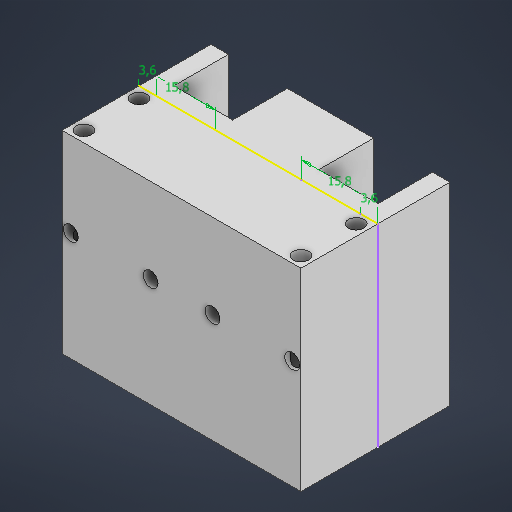
# Autodesk Inventor part: peça2
Saved by Autodesk Inventor 2026 (Build 300175000, 175)
## iProperties
Created: 2026-04-17
Part Number: peça2
Material: Genérico
Document SubType Name: Modeling
Designer: a2453266
Density: 1 g/cm^3
Appearance: Padrão
Author: a2453266
Autodesk Inventor part; units mm, degrees
ref_plane "YZ Plane" through (0, 0, 0) normal (1, 0, 0) x (0, 1, 0)
ref_plane "XZ Plane" through (0, 0, 0) normal (0, 1, 0) x (-1, 0, 0)
ref_plane "XY Plane" through (0, 0, 0) normal (0, 0, 1) x (1, 0, 0)
sketch "Esboço1" plane through (0, 0, 0) normal (0, 1, 0) x (-1, 0, 0)
  line L0 (0, 0) -> (-49.4, 0)
  line L1 (-49.4, 0) -> (-49.4, -15.9)
  line L2 (-49.4, -15.9) -> (0, -15.9)
  line L3 (0, -15.9) -> (0, 0)
  dimension "d0" = 49.4
  dimension "d1" = 15.9
  constraints: 8 end point, 2 parallel, 1 horizontal, 1 perpendicular
  measures "d0" distance of L2.end L1.end
  measures "d1" distance of L1.end L0.end
extrude "Extrusão1" add sketch "Esboço1" along normal blind 40
sketch "Esboço2" plane through (0, 40, 0) normal (0, 1, 0) x (1, 0, 0)
  line L0 (49.4, 15.9) -> (0, 15.9) projected
  line L1 (0, 15.9) -> (4.5, 15.9)
  line L2 (4.5, 15.9) -> (4.5, 11.4)
  line L3 (4.5, 11.4) -> (0, 11.4)
  line L4 (0, 11.4) -> (0, 15.9)
  line L5 (0, 0) -> (49.4, 0) projected
  line L6 (0, 0) -> (4.5, 0)
  line L7 (4.5, 0) -> (4.5, 4.5)
  line L8 (4.5, 4.5) -> (0, 4.5)
  line L9 (0, 4.5) -> (0, 0)
  line L10 (49.4, 0) -> (49.4, 15.9) projected
  line L11 (49.4, 15.9) -> (44.9, 15.9)
  line L12 (44.9, 15.9) -> (44.9, 11.4)
  line L13 (44.9, 11.4) -> (49.4, 11.4)
  line L14 (49.4, 11.4) -> (49.4, 15.9)
  line L15 (49.4, 0) -> (44.9, 0)
  line L16 (44.9, 0) -> (44.9, 4.5)
  line L17 (44.9, 4.5) -> (49.4, 4.5)
  line L18 (49.4, 4.5) -> (49.4, 0)
  line L19 (2.25, 15.9) -> (2.25, 11.4)
  line L20 (2.25, 4.5) -> (2.25, 0)
  line L21 (47.15, 15.9) -> (47.15, 11.4)
  line L22 (47.15, 4.5) -> (47.15, 0)
  circle A0 centre (2.25, 13.65) radius 1.6
  circle A1 centre (2.25, 2.25) radius 1.6
  circle A2 centre (47.15, 13.65) radius 1.6
  circle A3 centre (47.15, 2.25) radius 1.6
  dimension "d4" = 4.5
  dimension "d5" = 4.5
  dimension "d6" = 4.5
  dimension "d7" = 4.5
  dimension "d8" = 4.5
  dimension "d9" = 4.5
  dimension "d10" = 4.5
  dimension "d11" = 4.5
  dimension "d12" = 3.2
  dimension "d13" = 3.2
  dimension "d14" = 3.2
  dimension "d15" = 3.2
  constraints: 40 end point, 12 midpoint, 8 parallel, 4 centre point, 4 horizontal, 4 perpendicular
  measures "d4" distance of L2.end L3.end
  measures "d5" distance of L1.end L2.end
  measures "d6" distance of L8.end L7.end
  measures "d7" distance of L7.end L6.end
  measures "d8" distance of L13.end L12.end
  measures "d9" distance of L12.end L11.end
  measures "d10" distance of L16.end L17.end
  measures "d11" distance of L15.end L16.end
  measures "d12" diameter of A0
  measures "d13" diameter of A1
  measures "d14" diameter of A2
  measures "d15" diameter of A3
extrude "Extrusão2" cut sketch "Esboço2" against normal blind 40 contours A2 L21 | L21 A2 | A3 L22 | L22 A3 | A0 L19 | L19 A0 | A1 L20 | L20 A1
sketch "Esboço3" plane through (49.4, 0, -15.9) normal (0, 0, -1) x (-1, 0, 0)
  line L0 (49.4, 40) -> (0, 40) projected
  line L1 (49.4, 0) -> (33.6, 0)
  line L2 (33.6, 0) -> (33.6, 40)
  line L3 (33.6, 40) -> (49.4, 40)
  line L4 (49.4, 40) -> (49.4, 0)
  line L5 (0, 0) -> (15.8, 0)
  line L6 (15.8, 0) -> (15.8, 40)
  line L7 (15.8, 40) -> (0, 40)
  line L8 (0, 40) -> (0, 0)
  line L9 (33.6, 0) -> (15.8, 0)
  line L10 (15.8, 0) -> (15.8, 40)
  line L11 (15.8, 40) -> (33.6, 40)
  line L12 (33.6, 40) -> (33.6, 0)
  line L13 (49.4, 0) -> (45.8, 0)
  line L14 (45.8, 0) -> (45.8, 40)
  line L15 (45.8, 40) -> (49.4, 40)
  line L16 (49.4, 40) -> (49.4, 0)
  line L17 (0, 0) -> (3.6, 0)
  line L18 (3.6, 0) -> (3.6, 40)
  line L19 (3.6, 40) -> (0, 40)
  line L20 (0, 40) -> (0, 0)
  point P0 (3.6, 0)
  point P1 (3.6, 40)
  dimension "d18" = 15.8
  dimension "d19" = 15.8
  dimension "d24" = 3.6
  dimension "d25" = 3.6
  constraints: 40 end point, 10 parallel, 5 horizontal, 5 perpendicular, 5 point on line
  measures "d18" distance of L2.end L3.end
  measures "d19" distance of L7.end L6.end
  measures "d24" distance of L14.end L15.end
  measures "d25" distance of L19.end L18.end
extrude "Extrusão3" add sketch "Esboço3" along normal blind 14.9 contours L2 L9 L6 L0
extrude "Extrusão4" add sketch "Esboço3" along normal blind 3.6 contours L4 L1 L14 L0 | L14 L1 L2 L0 | L6 L5 L18 L0 | L18 L5 L8 L0
extrude "Extrusão5" add sketch "Esboço3" along normal blind 14.9 contours L4 L1 L14 L0 | L18 L5 L8 L0
sketch "Esboço4" plane through (49.4, 0, -30.8) normal (0, 0, -1) x (-1, 0, 0)
  point P0 (49.4, 0)
sketch "Esboço5" plane through (49.4, 0, -30.8) normal (0, 0, -1) x (-1, 0, 0)
  line L0 (15.8, 40) -> (15.8, 0) projected
  line L1 (33.6, 0) -> (33.6, 40) projected
  line L2 (15.8, 40) -> (33.6, 40)
  line L3 (33.6, 40) -> (33.6, 20)
  line L4 (33.6, 20) -> (15.8, 20)
  line L5 (15.8, 20) -> (15.8, 40)
  line L6 (15.8, 20) -> (33.6, 20)
  line L7 (33.6, 20) -> (33.6, 0)
  line L8 (33.6, 0) -> (15.8, 0)
  line L9 (15.8, 0) -> (15.8, 20)
  line L10 (15.8, 20) -> (33.6, 20)
  line L11 (33.6, 20) -> (33.6, 25)
  line L12 (33.6, 25) -> (15.8, 25)
  line L13 (15.8, 25) -> (15.8, 20)
  line L14 (15.8, 20) -> (20.8, 20)
  line L15 (20.8, 20) -> (20.8, 25)
  line L16 (20.8, 25) -> (15.8, 25)
  line L17 (15.8, 25) -> (15.8, 20)
  line L18 (33.6, 20) -> (28.6, 20)
  line L19 (28.6, 20) -> (28.6, 25)
  line L20 (28.6, 25) -> (33.6, 25)
  line L21 (33.6, 25) -> (33.6, 20)
  line L22 (18.3, 25) -> (18.3, 20)
  circle A0 centre (18.3, 22.5) radius 1.55
  line L23 (31.1, 25) -> (31.1, 20)
  circle A1 centre (31.1, 22.5) radius 1.55
  line L24 (0, 40) -> (0, 0) projected
  line L25 (15.8, 25) -> (0, 25)
  line L26 (0, 25) -> (0, 20)
  line L27 (0, 20) -> (15.8, 20)
  line L28 (15.8, 20) -> (15.8, 25)
  line L29 (33.6, 25) -> (49.4, 25)
  line L30 (49.4, 25) -> (49.4, 20)
  line L31 (49.4, 20) -> (33.6, 20)
  line L32 (33.6, 20) -> (33.6, 25)
  line L33 (0, 22.5) -> (3.6, 22.5)
  line L34 (3.6, 40) -> (3.6, 0) projected
  line L35 (49.4, 22.5) -> (45.8, 22.5)
  line L36 (45.8, 0) -> (45.8, 40) projected
  circle A2 centre (1.8, 22.5) radius 1.55
  circle A3 centre (47.6, 22.5) radius 1.55
  point P0 (49.4, 0)
  dimension "d28" = 20
  dimension "d29" = 5
  dimension "d30" = 5
  dimension "d31" = 5
  dimension "d32" = 5
  dimension "d33" = 3.1
  dimension "d34" = 3.1
  dimension "d35" = 3.1
  dimension "d36" = 3.1
  constraints: 64 end point, 14 parallel, 12 midpoint, 9 horizontal, 7 perpendicular, 4 centre point, 4 point on line
  measures "d28" distance of L2.end L3.end
  measures "d29" distance of L11.end L10.end
  measures "d30" distance of L16.end L15.end
  measures "d31" distance of L19.end L20.end
  measures "d32" distance of L18.end L19.end
  measures "d33" diameter of A0
  measures "d34" diameter of A1
  measures "d35" diameter of A2
  measures "d36" diameter of A3
extrude "Extrusão6" cut sketch "Esboço5" against normal through all contours A0 L22 | L22 A0 | A2 L33 | L33 A2 | A1 L23 | L23 A1 | A3 L35 | L35 A3
